Autodesk Fusion 360 part; units mm, degrees
(part 3 of 3)
sketch "sketch 8887" plane through (0, 0, 10) normal (0, 0, 1) x (-1, 0, 0)
  line L0 (-24.45, 23.2877) -> (-24.45, 24.3)
  line L1 (-21.3995, 23.2877) -> (-24.45, 23.2877)
  line L2 (-24.45, 22.5092) -> (-21.3995, 23.2877)
  line L3 (-24.45, 21.5929) -> (-24.45, 22.5092)
  line L4 (-21.3995, 20.813) -> (-24.45, 21.5929)
  line L5 (-24.45, 20.813) -> (-21.3995, 20.813)
  line L6 (-24.45, 19.8007) -> (-24.45, 20.813)
  line L7 (-20.45, 19.8007) -> (-24.45, 19.8007)
  line L8 (-20.45, 21.4252) -> (-20.45, 19.8007)
  line L9 (-22.8838, 22.0476) -> (-20.45, 21.4252)
  line L10 (-20.45, 22.6745) -> (-22.8838, 22.0476)
  line L11 (-20.45, 24.3) -> (-20.45, 22.6745)
  line L12 (-24.45, 24.3) -> (-20.45, 24.3)
  line L13 (-14.95, 19.195) -> (-14.95, 20.3819)
  line L14 (-13.8368, 19.195) -> (-14.95, 19.195)
  line L15 (-13.8368, 20.3819) -> (-13.8368, 19.195)
  line L16 (-14.95, 20.3819) -> (-13.8368, 20.3819)
  spline S0 degree 2 poles (-1.5721, 17.6288) (-1.5721, 17.8252) (-1.6908, 17.948) knots 0 0 0 1 1 1
  spline S1 degree 2 poles (-1.6812, 17.3286) (-1.5721, 17.4378) (-1.5721, 17.6288) knots 0 0 0 1 1 1
  spline S2 degree 2 poles (-1.9732, 17.2195) (-1.7904, 17.2195) (-1.6812, 17.3286) knots 0 0 0 1 1 1
  spline S3 degree 2 poles (-2.3033, 17.3655) (-2.1642, 17.2195) (-1.9732, 17.2195) knots 0 0 0 1 1 1
  spline S4 degree 2 poles (-2.4425, 17.7297) (-2.4425, 17.5115) (-2.3033, 17.3655) knots 0 0 0 1 1 1
  spline S5 degree 2 poles (-2.4289, 17.8744) (-2.4425, 17.7816) (-2.4425, 17.7297) knots 0 0 0 1 1 1
  line L17 (-3.2229, 17.9317) -> (-2.4289, 17.8744)
  spline S6 degree 2 poles (-3.1574, 17.5715) (-3.1574, 17.7025) (-3.2229, 17.9317) knots 0 0 0 1 1 1
  spline S7 degree 2 poles (-3.3102, 17.1827) (-3.1574, 17.3259) (-3.1574, 17.5715) knots 0 0 0 1 1 1
  spline S8 degree 2 poles (-3.7413, 17.0394) (-3.463, 17.0394) (-3.3102, 17.1827) knots 0 0 0 1 1 1
  spline S9 degree 2 poles (-4.1778, 17.1881) (-4.0141, 17.0394) (-3.7413, 17.0394) knots 0 0 0 1 1 1
  spline S10 degree 2 poles (-4.3415, 17.5606) (-4.3415, 17.3368) (-4.1778, 17.1881) knots 0 0 0 1 1 1
  spline S11 degree 2 poles (-4.2119, 17.9112) (-4.3415, 17.7734) (-4.3415, 17.5606) knots 0 0 0 1 1 1
  spline S12 degree 2 poles (-3.7467, 18.1145) (-4.0823, 18.049) (-4.2119, 17.9112) knots 0 0 0 1 1 1
  line L18 (-3.8941, 19.225) -> (-3.7467, 18.1145)
  spline S13 degree 2 poles (-4.5148, 18.9126) (-4.2679, 19.1158) (-3.8941, 19.225) knots 0 0 0 1 1 1
  spline S14 degree 2 poles (-4.89, 18.3941) (-4.7617, 18.7093) (-4.5148, 18.9126) knots 0 0 0 1 1 1
  spline S15 degree 2 poles (-5.0182, 17.5333) (-5.0182, 18.079) (-4.89, 18.3941) knots 0 0 0 1 1 1
  spline S16 degree 2 poles (-4.845, 16.6302) (-5.0182, 16.9739) (-5.0182, 17.5333) knots 0 0 0 1 1 1
  spline S17 degree 2 poles (-4.3511, 16.1035) (-4.6717, 16.2864) (-4.845, 16.6302) knots 0 0 0 1 1 1
  spline S18 degree 2 poles (-3.6812, 15.9207) (-4.0305, 15.9207) (-4.3511, 16.1035) knots 0 0 0 1 1 1
  spline S19 degree 2 poles (-3.2024, 16.0312) (-3.4029, 15.9207) (-3.6812, 15.9207) knots 0 0 0 1 1 1
  spline S20 degree 2 poles (-2.8791, 16.3409) (-3.0018, 16.1417) (-3.2024, 16.0312) knots 0 0 0 1 1 1
  spline S21 degree 2 poles (-2.7454, 16.6956) (-2.8027, 16.4637) (-2.8791, 16.3409) knots 0 0 0 1 1 1
  spline S22 degree 2 poles (-2.377, 16.2673) (-2.5871, 16.4091) (-2.7454, 16.6956) knots 0 0 0 1 1 1
  spline S23 degree 2 poles (-1.9077, 16.1254) (-2.1669, 16.1254) (-2.377, 16.2673) knots 0 0 0 1 1 1
  spline S24 degree 2 poles (-1.1737, 16.4746) (-1.4657, 16.1254) (-1.9077, 16.1254) knots 0 0 0 1 1 1
  spline S25 degree 2 poles (-0.8818, 17.607) (-0.8818, 16.8239) (-1.1737, 16.4746) knots 0 0 0 1 1 1
  spline S26 degree 2 poles (-1.1492, 18.6615) (-0.8818, 18.2891) (-0.8818, 17.607) knots 0 0 0 1 1 1
  spline S27 degree 2 poles (-1.9186, 19.1649) (-1.4166, 19.034) (-1.1492, 18.6615) knots 0 0 0 1 1 1
  line L19 (-2.1069, 18.1145) -> (-1.9186, 19.1649)
  spline S28 degree 2 poles (-1.6908, 17.948) (-1.8095, 18.0708) (-2.1069, 18.1145) knots 0 0 0 1 1 1
  line L20 (7.1598, 17.2823) -> (7.1598, 18.352)
  line L21 (7.1598, 18.352) -> (8.4186, 17.2823)
  line L22 (8.4186, 17.2823) -> (7.1598, 17.2823)
  line L23 (5.55, 16.3136) -> (5.55, 17.2823)
  line L24 (6.2976, 16.3136) -> (5.55, 16.3136)
  line L25 (6.2976, 15.8116) -> (6.2976, 16.3136)
  line L26 (7.1598, 15.8116) -> (6.2976, 15.8116)
  line L27 (7.1598, 16.3136) -> (7.1598, 15.8116)
  line L28 (9.6182, 16.3136) -> (7.1598, 16.3136)
  line L29 (9.6182, 17.2823) -> (9.6182, 16.3136)
  line L30 (7.2117, 19.3068) -> (9.6182, 17.2823)
  line L31 (6.2976, 19.3068) -> (7.2117, 19.3068)
  line L32 (6.2976, 17.2823) -> (6.2976, 19.3068)
  line L33 (5.55, 17.2823) -> (6.2976, 17.2823)
  line L34 (18.7635, 18.1472) -> (18.8999, 19.094)
  spline S29 degree 2 poles (18.9709, 17.9016) (18.9136, 18.0135) (18.7635, 18.1472) knots 0 0 0 1 1 1
  spline S30 degree 2 poles (19.05, 17.5906) (19.05, 17.7516) (18.9709, 17.9016) knots 0 0 0 1 1 1
  spline S31 degree 2 poles (18.8836, 17.184) (19.05, 17.3368) (19.05, 17.5906) knots 0 0 0 1 1 1
  spline S32 degree 2 poles (18.3597, 17.0312) (18.7171, 17.0312) (18.8836, 17.184) knots 0 0 0 1 1 1
  spline S33 degree 2 poles (17.8344, 17.1827) (18.0104, 17.0312) (18.3597, 17.0312) knots 0 0 0 1 1 1
  spline S34 degree 2 poles (17.6585, 17.566) (17.6585, 17.3341) (17.8344, 17.1827) knots 0 0 0 1 1 1
  spline S35 degree 2 poles (17.799, 17.9235) (17.6585, 17.7734) (17.6585, 17.566) knots 0 0 0 1 1 1
  spline S36 degree 2 poles (18.2096, 18.1145) (17.9395, 18.0735) (17.799, 17.9235) knots 0 0 0 1 1 1
  line L35 (18.0868, 19.2386) -> (18.2096, 18.1145)
  spline S37 degree 2 poles (17.6175, 19.034) (17.8058, 19.1568) (18.0868, 19.2386) knots 0 0 0 1 1 1
  spline S38 degree 2 poles (17.2806, 18.7134) (17.4293, 18.9112) (17.6175, 19.034) knots 0 0 0 1 1 1
  spline S39 degree 2 poles (17.0568, 18.2332) (17.1319, 18.5156) (17.2806, 18.7134) knots 0 0 0 1 1 1
  spline S40 degree 2 poles (16.9818, 17.5551) (16.9818, 17.9508) (17.0568, 18.2332) knots 0 0 0 1 1 1
  spline S41 degree 2 poles (17.1701, 16.6506) (16.9818, 17.004) (16.9818, 17.5551) knots 0 0 0 1 1 1
  spline S42 degree 2 poles (17.7158, 16.1049) (17.3583, 16.2973) (17.1701, 16.6506) knots 0 0 0 1 1 1
  spline S43 degree 2 poles (18.4606, 15.9126) (18.0732, 15.9126) (17.7158, 16.1049) knots 0 0 0 1 1 1
  spline S44 degree 2 poles (19.3747, 16.2864) (19.0118, 15.9126) (18.4606, 15.9126) knots 0 0 0 1 1 1
  spline S45 degree 2 poles (19.7376, 17.2604) (19.7376, 16.6602) (19.3747, 16.2864) knots 0 0 0 1 1 1
  spline S46 degree 2 poles (19.6939, 17.6192) (19.7376, 17.4378) (19.7376, 17.2604) knots 0 0 0 1 1 1
  spline S47 degree 2 poles (19.563, 17.9862) (19.6503, 17.8007) (19.6939, 17.6192) knots 0 0 0 1 1 1
  line L36 (20.1632, 17.8907) -> (19.563, 17.9862)
  line L37 (20.1632, 16.1035) -> (20.1632, 17.8907)
  line L38 (21.05, 16.1035) -> (20.1632, 16.1035)
  line L39 (21.05, 18.742) -> (21.05, 16.1035)
  line L40 (18.8999, 19.094) -> (21.05, 18.742)
  line L41 (17.05, 23.2877) -> (17.05, 24.3)
  line L42 (20.1005, 23.2877) -> (17.05, 23.2877)
  line L43 (17.05, 22.5092) -> (20.1005, 23.2877)
  line L44 (17.05, 21.5929) -> (17.05, 22.5092)
  line L45 (20.1005, 20.813) -> (17.05, 21.5929)
  line L46 (17.05, 20.813) -> (20.1005, 20.813)
  line L47 (17.05, 19.8007) -> (17.05, 20.813)
  line L48 (21.05, 19.8007) -> (17.05, 19.8007)
  line L49 (21.05, 21.4252) -> (21.05, 19.8007)
  line L50 (18.6162, 22.0476) -> (21.05, 21.4252)
  line L51 (21.05, 22.6745) -> (18.6162, 22.0476)
  line L52 (21.05, 24.3) -> (21.05, 22.6745)
  line L53 (17.05, 24.3) -> (21.05, 24.3)
  line L54 (5.55, 23.2877) -> (5.55, 24.3)
  line L55 (8.6005, 23.2877) -> (5.55, 23.2877)
  line L56 (5.55, 22.5092) -> (8.6005, 23.2877)
  line L57 (5.55, 21.5929) -> (5.55, 22.5092)
  line L58 (8.6005, 20.813) -> (5.55, 21.5929)
  line L59 (5.55, 20.813) -> (8.6005, 20.813)
  line L60 (5.55, 19.8007) -> (5.55, 20.813)
  line L61 (9.55, 19.8007) -> (5.55, 19.8007)
  line L62 (9.55, 21.4252) -> (9.55, 19.8007)
  line L63 (7.1162, 22.0476) -> (9.55, 21.4252)
  line L64 (9.55, 22.6745) -> (7.1162, 22.0476)
  line L65 (9.55, 24.3) -> (9.55, 22.6745)
  line L66 (5.55, 24.3) -> (9.55, 24.3)
  line L67 (-4.95, 23.2877) -> (-4.95, 24.3)
  line L68 (-1.8995, 23.2877) -> (-4.95, 23.2877)
  line L69 (-4.95, 22.5092) -> (-1.8995, 23.2877)
  line L70 (-4.95, 21.5929) -> (-4.95, 22.5092)
  line L71 (-1.8995, 20.813) -> (-4.95, 21.5929)
  line L72 (-4.95, 20.813) -> (-1.8995, 20.813)
  line L73 (-4.95, 19.8007) -> (-4.95, 20.813)
  line L74 (-0.95, 19.8007) -> (-4.95, 19.8007)
  line L75 (-0.95, 21.4252) -> (-0.95, 19.8007)
  line L76 (-3.3838, 22.0476) -> (-0.95, 21.4252)
  line L77 (-0.95, 22.6745) -> (-3.3838, 22.0476)
  line L78 (-0.95, 24.3) -> (-0.95, 22.6745)
  line L79 (-4.95, 24.3) -> (-0.95, 24.3)
  line L80 (-13.2365, 17.5851) -> (-13.1001, 18.5319)
  spline S48 degree 2 poles (-13.0291, 17.3396) (-13.0864, 17.4514) (-13.2365, 17.5851) knots 0 0 0 1 1 1
  spline S49 degree 2 poles (-12.95, 17.0285) (-12.95, 17.1895) (-13.0291, 17.3396) knots 0 0 0 1 1 1
  spline S50 degree 2 poles (-13.1164, 16.622) (-12.95, 16.7748) (-12.95, 17.0285) knots 0 0 0 1 1 1
  spline S51 degree 2 poles (-13.6403, 16.4692) (-13.2829, 16.4692) (-13.1164, 16.622) knots 0 0 0 1 1 1
  spline S52 degree 2 poles (-14.1656, 16.6206) (-13.9896, 16.4692) (-13.6403, 16.4692) knots 0 0 0 1 1 1
  spline S53 degree 2 poles (-14.3415, 17.004) (-14.3415, 16.772) (-14.1656, 16.6206) knots 0 0 0 1 1 1
  spline S54 degree 2 poles (-14.201, 17.3614) (-14.3415, 17.2113) (-14.3415, 17.004) knots 0 0 0 1 1 1
  spline S55 degree 2 poles (-13.7904, 17.5524) (-14.0605, 17.5115) (-14.201, 17.3614) knots 0 0 0 1 1 1
  line L81 (-13.9132, 18.6765) -> (-13.7904, 17.5524)
  spline S56 degree 2 poles (-14.3825, 18.4719) (-14.1942, 18.5947) (-13.9132, 18.6765) knots 0 0 0 1 1 1
  spline S57 degree 2 poles (-14.7194, 18.1513) (-14.5707, 18.3491) (-14.3825, 18.4719) knots 0 0 0 1 1 1
  spline S58 degree 2 poles (-14.9432, 17.6711) (-14.8681, 17.9535) (-14.7194, 18.1513) knots 0 0 0 1 1 1
  spline S59 degree 2 poles (-15.0182, 16.993) (-15.0182, 17.3887) (-14.9432, 17.6711) knots 0 0 0 1 1 1
  spline S60 degree 2 poles (-14.8299, 16.0885) (-15.0182, 16.4419) (-15.0182, 16.993) knots 0 0 0 1 1 1
  spline S61 degree 2 poles (-14.2842, 15.5428) (-14.6417, 15.7352) (-14.8299, 16.0885) knots 0 0 0 1 1 1
  spline S62 degree 2 poles (-13.5394, 15.3505) (-13.9268, 15.3505) (-14.2842, 15.5428) knots 0 0 0 1 1 1
  spline S63 degree 2 poles (-12.6253, 15.7243) (-12.9882, 15.3505) (-13.5394, 15.3505) knots 0 0 0 1 1 1
  spline S64 degree 2 poles (-12.2624, 16.6984) (-12.2624, 16.0981) (-12.6253, 15.7243) knots 0 0 0 1 1 1
  spline S65 degree 2 poles (-12.3061, 17.0572) (-12.2624, 16.8757) (-12.2624, 16.6984) knots 0 0 0 1 1 1
  spline S66 degree 2 poles (-12.437, 17.4241) (-12.3497, 17.2386) (-12.3061, 17.0572) knots 0 0 0 1 1 1
  line L82 (-11.8368, 17.3286) -> (-12.437, 17.4241)
  line L83 (-11.8368, 15.5415) -> (-11.8368, 17.3286)
  line L84 (-10.95, 15.5415) -> (-11.8368, 15.5415)
  line L85 (-10.95, 18.1799) -> (-10.95, 15.5415)
  line L86 (-13.1001, 18.5319) -> (-10.95, 18.1799)
  line L87 (-14.0441, 22.7011) -> (-14.0441, 20.9658)
  spline S67 degree 2 poles (-13.8013, 22.4351) (-13.8941, 22.5483) (-14.0441, 22.7011) knots 0 0 0 1 1 1
  spline S68 degree 2 poles (-13.4766, 21.9862) (-13.7085, 22.3218) (-13.8013, 22.4351) knots 0 0 0 1 1 1
  spline S69 degree 2 poles (-12.7454, 21.2072) (-13.0782, 21.4214) (-13.4766, 21.9862) knots 0 0 0 1 1 1
  spline S70 degree 2 poles (-12.0469, 20.993) (-12.4125, 20.993) (-12.7454, 21.2072) knots 0 0 0 1 1 1
  spline S71 degree 2 poles (-11.4261, 21.1799) (-11.7031, 20.993) (-12.0469, 20.993) knots 0 0 0 1 1 1
  spline S72 degree 2 poles (-11.0155, 21.6929) (-11.1492, 21.3668) (-11.4261, 21.1799) knots 0 0 0 1 1 1
  spline S73 degree 2 poles (-10.8818, 22.6056) (-10.8818, 22.019) (-11.0155, 21.6929) knots 0 0 0 1 1 1
  spline S74 degree 2 poles (-11.0223, 23.4855) (-10.8818, 23.1677) (-10.8818, 22.6056) knots 0 0 0 1 1 1
  spline S75 degree 2 poles (-11.4261, 23.978) (-11.1628, 23.8034) (-11.0223, 23.4855) knots 0 0 0 1 1 1
  spline S76 degree 2 poles (-12.1587, 24.2181) (-11.6894, 24.1527) (-11.4261, 23.978) knots 0 0 0 1 1 1
  line L88 (-12.2488, 23.1049) -> (-12.1587, 24.2181)
  spline S77 degree 2 poles (-11.7767, 22.9235) (-11.9104, 23.0585) (-12.2488, 23.1049) knots 0 0 0 1 1 1
  spline S78 degree 2 poles (-11.643, 22.5756) (-11.643, 22.7884) (-11.7767, 22.9235) knots 0 0 0 1 1 1
  spline S79 degree 2 poles (-11.7726, 22.2359) (-11.643, 22.3709) (-11.643, 22.5756) knots 0 0 0 1 1 1
  spline S80 degree 2 poles (-12.0851, 22.1008) (-11.9023, 22.1008) (-11.7726, 22.2359) knots 0 0 0 1 1 1
  spline S81 degree 2 poles (-12.4425, 22.2372) (-12.2542, 22.1008) (-12.0851, 22.1008) knots 0 0 0 1 1 1
  spline S82 degree 2 poles (-12.9937, 22.8621) (-12.6308, 22.3737) (-12.4425, 22.2372) knots 0 0 0 1 1 1
  spline S83 degree 2 poles (-14.0209, 23.9521) (-13.5857, 23.6615) (-12.9937, 22.8621) knots 0 0 0 1 1 1
  spline S84 degree 2 poles (-14.95, 24.3) (-14.4561, 24.2427) (-14.0209, 23.9521) knots 0 0 0 1 1 1
  line L89 (-14.95, 20.9658) -> (-14.95, 24.3)
  line L90 (-14.0441, 20.9658) -> (-14.95, 20.9658)
  line L91 (-23.5441, 17.6752) -> (-23.5441, 15.9398)
  spline S85 degree 2 poles (-23.3013, 17.4091) (-23.3941, 17.5224) (-23.5441, 17.6752) knots 0 0 0 1 1 1
  spline S86 degree 2 poles (-22.9766, 16.9603) (-23.2085, 17.2959) (-23.3013, 17.4091) knots 0 0 0 1 1 1
  spline S87 degree 2 poles (-22.2454, 16.1813) (-22.5782, 16.3955) (-22.9766, 16.9603) knots 0 0 0 1 1 1
  spline S88 degree 2 poles (-21.5469, 15.9671) (-21.9125, 15.9671) (-22.2454, 16.1813) knots 0 0 0 1 1 1
  spline S89 degree 2 poles (-20.9261, 16.154) (-21.2031, 15.9671) (-21.5469, 15.9671) knots 0 0 0 1 1 1
  spline S90 degree 2 poles (-20.5155, 16.667) (-20.6492, 16.3409) (-20.9261, 16.154) knots 0 0 0 1 1 1
  spline S91 degree 2 poles (-20.3818, 17.5797) (-20.3818, 16.993) (-20.5155, 16.667) knots 0 0 0 1 1 1
  spline S92 degree 2 poles (-20.5223, 18.4596) (-20.3818, 18.1417) (-20.3818, 17.5797) knots 0 0 0 1 1 1
  spline S93 degree 2 poles (-20.9261, 18.9521) (-20.6628, 18.7775) (-20.5223, 18.4596) knots 0 0 0 1 1 1
  spline S94 degree 2 poles (-21.6587, 19.1922) (-21.1894, 19.1267) (-20.9261, 18.9521) knots 0 0 0 1 1 1
  line L92 (-21.7488, 18.079) -> (-21.6587, 19.1922)
  spline S95 degree 2 poles (-21.2767, 17.8975) (-21.4104, 18.0326) (-21.7488, 18.079) knots 0 0 0 1 1 1
  spline S96 degree 2 poles (-21.143, 17.5497) (-21.143, 17.7625) (-21.2767, 17.8975) knots 0 0 0 1 1 1
  spline S97 degree 2 poles (-21.2726, 17.21) (-21.143, 17.345) (-21.143, 17.5497) knots 0 0 0 1 1 1
  spline S98 degree 2 poles (-21.5851, 17.0749) (-21.4023, 17.0749) (-21.2726, 17.21) knots 0 0 0 1 1 1
  spline S99 degree 2 poles (-21.9425, 17.2113) (-21.7542, 17.0749) (-21.5851, 17.0749) knots 0 0 0 1 1 1
  spline S100 degree 2 poles (-22.4937, 17.8362) (-22.1308, 17.3477) (-21.9425, 17.2113) knots 0 0 0 1 1 1
  spline S101 degree 2 poles (-23.5209, 18.9262) (-23.0857, 18.6356) (-22.4937, 17.8362) knots 0 0 0 1 1 1
  spline S102 degree 2 poles (-24.45, 19.2741) (-23.9561, 19.2168) (-23.5209, 18.9262) knots 0 0 0 1 1 1
  line L93 (-24.45, 15.9398) -> (-24.45, 19.2741)
  line L94 (-23.5441, 15.9398) -> (-24.45, 15.9398)
extrude "Extrude - Labels Only" add sketch "sketch 3553" sketch "sketch 8887" along normal blind 0.4 of sketch 2 makes body 1 at (-8.0531, -9.9025, 10) makes body 2 at (11.9469, -9.9025, 10) makes body 3 at (11.4172, -11.2623, 10) makes body 4 at (-11.8157, -9.574, 10) makes body 5 at (8.1843, -9.574, 10) makes body 6 at (-4.3542, 18.3859, 10) makes body 7 at (-9.9641, 21.869, 10) makes body 8 at (17.4172, 19.2836, 10) makes body 9 at (-4.3542, 21.6472, 10) makes body 10 at (5.4172, 22.4733, 10) makes body 11 at (15.6458, 21.6758, 10) makes body 12 at (13.4172, 19.2836, 10) makes body 13 at (9.9957, 18.7588, 10) makes body 14 at (-0.3542, 18.3859, 10) makes body 15 at (18.1843, 21.0006, 10) makes body 16 at (-18.0541, 18.6247, 10) makes body 17 at (-14.0541, 18.6247, 10) makes body 18 at (-6.3542, -12.1313, 10) makes body 19 at (7.9957, -11.7441, 10) makes body 20 at (-19.9641, -8.3785, 10) makes body 21 at (-12.0541, -11.6514, 10) makes body 22 at (15.4172, -11.3602, 10) makes body 23 at (15.4172, -8.0989, 10) makes body 24 at (-4.5828, -8.0989, 10) makes body 25 at (-14.3542, -8.8557, 10) makes body 26 at (1.6458, -12.1313, 10) makes body 27 at (20.0359, -8.3785, 10) makes body 28 at (5.6458, -8.8557, 10) makes body 29 at (-14.5828, 22.2464, 10) makes body 30 at (-21.8157, 17.6343, 10) makes body 31 at (21.9469, 20.5838, 10) makes body 32 at (5.9957, 18.7588, 10) makes body 33 at (-1.8157, 20.9719, 10) makes body 34 at (10.0359, 22.0958, 10) makes body 35 at (1.9957, 18.7588, 10) makes body 36 at (1.9469, 20.5718, 10) makes body 37 at (21.4708, 17.4994, 10) makes body 38 at (-10.0541, 18.6247, 10) makes body 39 at (-18.0531, 20.345, 10) makes body 40 at (-24.5828, -8.0989, 10) makes body 41 at (-2.3542, -12.2292, 10) makes body 42 at (0.0359, -8.3785, 10) makes body 43 at (-16.0541, -11.6085, 10) makes body 44 at (3.9957, -11.7011, 10) makes body 45 at (19.4172, -11.2623, 10) makes body 46 at (14.648, -22.6556, 10) makes body 47 at (2.5998, -23.9626, 10) makes body 48 at (-19.4002, -23.9626, 10) makes body 49 at (-8.3989, -16.6365, 10) makes body 50 at (14.2078, -19.5906, 10) makes body 51 at (22.0998, -23.9626, 10) makes body 52 at (2.7623, -17.1544, 10) makes body 53 at (-19.8376, -18.6074, 10) makes body 54 at (-7.9002, -23.9626, 10) makes body 55 at (12.1624, -18.0453, 10) makes body 56 at (24.148, -17.6297, 10)
